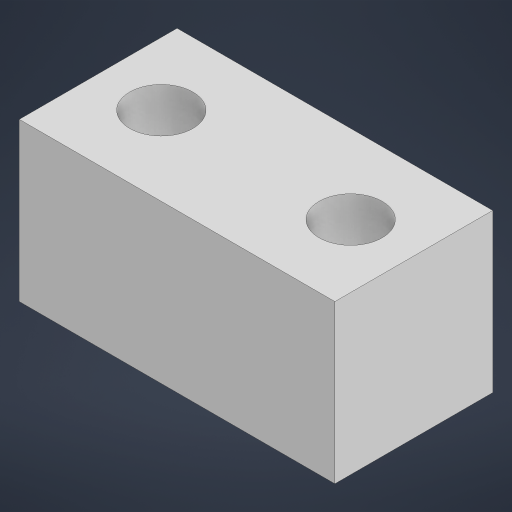
# Autodesk Inventor part: link
Saved by Autodesk Inventor 2024.3 (Build 283343000, 343)
## iProperties
Created: 2024-09-28
Part Number: link
Material: Generic
Document SubType Name: Modeling
Designer: sam
Density: 1 g/cm^3
Appearance: Default
Author: sam
Autodesk Inventor part; units mm, degrees
ref_plane "YZ Plane" through (0, 0, 0) normal (1, 0, 0) x (0, 1, 0)
ref_plane "XZ Plane" through (0, 0, 0) normal (0, 1, 0) x (-1, 0, 0)
ref_plane "XY Plane" through (0, 0, 0) normal (0, 0, 1) x (1, 0, 0)
sketch "Sketch1" plane through (0, 0, 0) normal (0, 1, 0) x (-1, 0, 0)
  line L0 (-5, -2.5) -> (5, -2.5)
  line L1 (5, 2.5) -> (5, 2.5)
  line L2 (5, 2.5) -> (-5, 2.5)
  line L3 (-5, 2.5) -> (-5, 2.5)
  line L4 (-5, -2.5) -> (5, 2.5) construction
  line L5 (5, -2.5) -> (-5, 2.5) construction
  circle A0 centre (3, 0) radius 1
  circle A1 centre (-3, 0) radius 1
  line L6 (5, 2.5) -> (5, -2.5)
  line L7 (-5, 2.5) -> (-5, -2.5)
  point P0 (0, 0)
  dimension "d1" = 10
  dimension "d3" = 2
  dimension "d4" = 2
  dimension "d5" = 2
  dimension "d6" = 2
  dimension "d7" = 2.5
  dimension "d8" = 2.5
  dimension "d12" = 5
  constraints: 16 end point, 4 midpoint, 2 centre point, 2 parallel, 2 perpendicular, 2 point on line, 1 horizontal, 1 vertical
  measures "d1" distance between parallel lines of L3 L1
  measures "d3" diameter of A0
  measures "d4" diameter of A1
  measures "d5" distance from line of L3 A1.centre
  measures "d6" distance from line of L1 A0.centre
  measures "d7" distance from line of L2 A1.centre
  measures "d8" distance from line of L2 A0.centre
  measures "d12" distance between parallel lines of L0 L2
extrude "Extrusion1" add sketch "Sketch1" along normal blind 5
body "Solid1"
